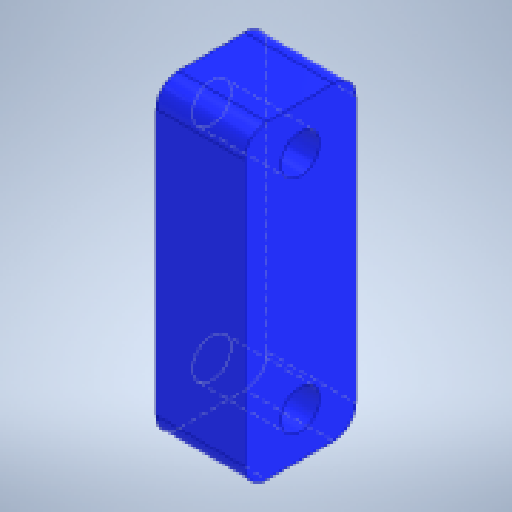
# Autodesk Inventor part: filler_side_fix
Saved by Autodesk Inventor 2025 (Build 290162000, 162)
## iProperties
Created: 2025-02-24
Part Number: filler_side_fix
Material: ABS プラスチック
Document SubType Name: Modeling
Designer: Zhopa
Density: 1.06 g/cm^3
Appearance: 青 - 壁塗料 - 光沢
Mass: 2.18211 g
Surface Area: 12.7111 cm^2
Volume: 2.05859 cm^3
Author: Zhopa
Autodesk Inventor part; units mm, degrees
ref_plane "YZ Plane" through (0, 0, 0) normal (1, 0, 0) x (0, 1, 0)
ref_plane "XZ Plane" through (0, 0, 0) normal (0, 1, 0) x (-1, 0, 0)
ref_plane "XY Plane" through (0, 0, 0) normal (0, 0, 1) x (1, 0, 0)
sketch "Sketch1" plane through (0, 0, 0) normal (1, 0, 0) x (0, 1, 0)
  line L0 (-14, -5) -> (14, -5)
  line L1 (14, -5) -> (14, 5)
  line L2 (14, 5) -> (-14, 5)
  line L3 (-14, 5) -> (-14, -5)
  line L4 (-14, -5) -> (14, 5) construction
  line L5 (14, -5) -> (-14, 5) construction
  circle A0 centre (10, 0) radius 1.75
  circle A1 centre (-10, 0) radius 1.75
  point P0 (0, 0)
  dimension "d0" = 10
  dimension "d1" = 28
  dimension "d2" = 4
  dimension "d3" = 4
  dimension "d4" = 3.5
  dimension "d5" = 3.5
  constraints: 12 end point, 2 centre point, 2 coincident, 2 midpoint, 2 parallel, 1 horizontal, 1 perpendicular
  measures "d0" distance of L1.end L0.end
  measures "d1" distance of L0.start L0.end
  measures "d2" distance from line of point (10, 0) L1
  measures "d3" distance from line of L3 point (-10, 0)
  measures "d4" diameter of A0
  measures "d5" diameter of A1
extrude "Extrusion1" add sketch "Sketch1" along normal blind 8
fillet "Fillet1" radius 2 4 edges at (4, 14, 5) (4, 14, -5) (4, -14, -5) (4, -14, 5)
body "Solid1"
